# Autodesk Inventor part: Zahnriemen
Saved by Autodesk Inventor 2016 (Build 200138000, 138)
## iProperties
Created: 2015-08-24
Part Number: Zahnriemen
Material: Rubber
Document SubType Name: Modeling
Designer: 4ndreas
Density: 1 g/cm^3
Appearance: Rubber - Black - Version 1.1
CustomPartVersion: 1
Author: 4ndreas
Autodesk Inventor part; units mm, degrees
sketch "Skizzenpfad" plane through (0, 0, 0) normal (0, 0, 1) x (1, 0, 0)
  arc A0 (24.2749, -23.1538) -> (-23.0321, -24.0729) centre (0, 8.3719) ccw
  arc A1 (7.4854, -36.0818) -> (5.0602, -43.6691) centre (11.756, -41.6281) ccw
  arc A2 (-11.963, -66.3767) -> (12.1791, -67.0232) centre (0, -70.7357) ccw
  arc A3 (-3.8183, -44.0246) -> (-6.3432, -35.9201) centre (-10.3952, -41.6281) ccw
  line L0 (-6.3432, -35.9201) -> (-23.0321, -24.0729)
  line L1 (24.2749, -23.1538) -> (7.4854, -36.0818)
  line L2 (5.0602, -43.6691) -> (12.1791, -67.0232)
  line L3 (-11.963, -66.3767) -> (-3.8183, -44.0246)
  constraints: 8 end point, 8 point on circle, 4 centre point
ref_plane "Querschnittsebene" through (-23.0321, -24.0729, 0) normal (0.8154, -0.5789, 0) x (0, 0, 1)
ref_plane "Arbeitsebene2" through (0, 8.3719, 0) normal (-1, 0, 0) x (0, 0, 1)
ref_plane "Arbeitsebene3" through (0, -70.7357, 0) normal (-0.136, 0.9907, 0) x (0, 0, 1)
sketch "Querschnitt" plane through (-23.0321, -24.0729, 0) normal (0.8154, -0.5789, 0) x (0, 0, 1)
  line L0 (-8, 0.5) -> (8, 0.5)
  line L1 (8, 0.5) -> (8, -0.5)
  line L2 (8, -0.5) -> (-8, -0.5)
  line L3 (-8, -0.5) -> (-8, 0.5)
  line L4 (-8, 0) -> (8, 0) construction
  point P0 (0, 0)
  point P1 (0, 0)
  dimension "d0" = 16
  dimension "d4" = 0.5
  dimension "d5" = 0.5
  constraints: 10 end point, 3 midpoint, 2 parallel, 1 coincident, 1 horizontal, 1 perpendicular, 1 other
  measures "d0" distance between parallel lines of L1 L3
  measures "d4" distance between parallel lines of L2 L4
  measures "d5" distance between parallel lines of L4 L0
sweep "Riemen" add profiles "Querschnitt" path "Skizzenpfad"
equation "\"d0\" = da_B"
equation "\"d4\" = da_a"
equation "\"d5\" = da_a2"
equation "\"da_B\" = 16"
equation "\"da_pb\" = 5"
equation "\"da_L\" = 355"
equation "\"da_a\" = 0.5"
equation "\"da_S\" = 2.65"
equation "\"da_Beta\" = 20deg"
equation "\"da_Ht\" = 1.2"
equation "\"da_H\" = 2.2"
equation "\"da_a2\" = 0.5"
body "Solid1"
